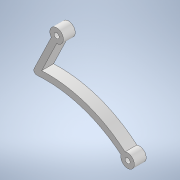
# Autodesk Inventor part: leg_link_3
Saved by Autodesk Inventor 2020 (Build 240168000, 168)
## iProperties
Created: 2020-12-12
Part Number: leg_link_3
Material: Generic
Document SubType Name: Modeling
Designer: Shuang Peng
Density: 1 g/cm^3
Appearance: Default
Author: Shuang Peng
Autodesk Inventor part; units mm, degrees
ref_plane "YZ Plane" through (0, 0, 0) normal (1, 0, 0) x (0, 1, 0)
ref_plane "XZ Plane" through (0, 0, 0) normal (0, 1, 0) x (-1, 0, 0)
ref_plane "XY Plane" through (0, 0, 0) normal (0, 0, 1) x (1, 0, 0)
sketch "Sketch1" plane through (0, 0, 0) normal (0, 0, 1) x (1, 0, 0)
  circle A0 centre (9.3299, 6.9995) radius 4
  line L0 (9.3299, 6.9995) -> (-2.3913, -17.3236)
  circle A1 centre (51.2129, -35.9635) radius 4
  line L1 (9.3299, 6.9995) -> (-2.3913, -17.3236) construction
  line L2 (7.7534, 7.7592) -> (-3.9678, -16.5639)
  line L3 (-0.8148, -18.0833) -> (10.9064, 6.2398)
  arc A2 (10.9064, 6.2398) -> (7.7534, 7.7592) centre (9.3299, 6.9995) ccw
  arc A3 (-3.9678, -16.5639) -> (-0.8148, -18.0833) centre (-2.3913, -17.3236) ccw
  arc A4 (-2.543, -15.5802) -> (-2.2396, -19.067) centre (-2.3913, -17.3236) ccw
  arc A5 (49.9598, -37.1851) -> (52.466, -34.7419) centre (51.2129, -35.9635) ccw
  arc A6 (49.9598, -37.1851) -> (-2.2396, -19.067) centre (2.7702, -88.8875) ccw
  arc A7 (52.466, -34.7419) -> (-2.543, -15.5802) centre (4.0227, -85.2716) ccw
  point P0 (0, 0)
  point P1 (3.4693, -5.1621)
  point P2 (47.3514, -34.9198)
  point P3 (49.7255, -32.2503)
  point P4 (0.4973, -15.3604)
  point P5 (9.3449, 2.9995)
  point P6 (6.1919, 4.5189)
  point P7 (-2.2396, -19.067)
  dimension "d0" = 8
  dimension "d1" = 27
  dimension "d3" = 8
  dimension "d4" = 3.5
  dimension "d6" = 3.5
  dimension "d7" = 70
  dimension "d8" = 70
  constraints: 12 point on circle, 10 end point, 8 centre point, 4 tangent, 2 coincident, 2 equal length, 1 midpoint, 2 other
  measures "d0" diameter of A0
  measures "d1" distance of L0.start L0.end
  measures "d3" diameter of A1
  measures "d4" diameter of A3
  measures "d6" diameter of A5
  measures "d7" radius of A6
  measures "d8" radius of A7
extrude "Extrusion1" add sketch "Sketch1" along normal blind 7
sketch "Sketch2" plane through (0, 0, 7) normal (0, 0, 1) x (1, 0, 0)
  line L0 (0.4973, -15.3604) -> (9.3449, 2.9995) projected
  arc A0 (9.3449, 2.9995) -> (6.1919, 4.5189) centre (9.3299, 6.9995) ccw projected
  line L1 (6.1919, 4.5189) -> (-3.9678, -16.5639) projected
  arc A1 (-3.9678, -16.5639) -> (-2.2396, -19.067) centre (-2.3913, -17.3236) ccw projected
  arc A2 (47.3514, -34.9198) -> (-2.2396, -19.067) centre (2.7702, -88.8875) ccw projected
  arc A3 (47.3514, -34.9198) -> (49.7255, -32.2503) centre (51.2129, -35.9635) ccw projected
  arc A4 (49.7255, -32.2503) -> (0.4973, -15.3604) centre (4.0227, -85.2716) ccw projected
  point P0 (0, 0)
hole "Hole1" at (51.2129, -35.9635, 7) at (9.3299, 6.9995, 7) direction (0, 0, -1) diameter 3 depth 8
sketch "Sketch3" plane through (0, 0, 0) normal (0, 0, -1) x (-1, 0, 0)
  circle A0 centre (-51.2129, -35.9635) radius 1.5 projected
  circle A1 centre (-9.3299, 6.9995) radius 1.5 projected
  line L0 (-0.4973, -15.3604) -> (-9.3449, 2.9995) projected
  arc A2 (-0.4973, -15.3604) -> (-49.7255, -32.2503) centre (-4.0227, -85.2716) ccw projected
  arc A3 (-49.7255, -32.2503) -> (-47.3514, -34.9198) centre (-51.2129, -35.9635) ccw projected
  arc A4 (2.2396, -19.067) -> (-47.3514, -34.9198) centre (-2.7702, -88.8875) ccw projected
  arc A5 (2.2396, -19.067) -> (3.9678, -16.5639) centre (2.3913, -17.3236) ccw projected
  line L1 (-6.1919, 4.5189) -> (3.9678, -16.5639) projected
  arc A6 (-6.1919, 4.5189) -> (-9.3449, 2.9995) centre (-9.3299, 6.9995) ccw projected
  circle A7 centre (-9.3299, 6.9995) radius 4
  circle A8 centre (-51.2129, -35.9635) radius 4
  point P0 (0, 0)
  point P1 (-49.7255, -32.2503)
  dimension "d18" = 8
  dimension "d19" = 8
  constraints: 2 centre point, 2 coincident
  measures "d18" diameter of A7
  measures "d19" diameter of A8
extrude "Extrusion2" cut sketch "Sketch3" against normal blind 2 contours L0 A7 L1 A5 A4 A8 A2
fillet "Fillet1" radius 2 6 edges at (47.3514, -34.9198, 4.5) (48.2239, -33.3053, 2) (49.7255, -32.2503, 4.5) (9.3449, 2.9995, 4.5) (7.5934, 3.3961, 2) (6.1919, 4.5189, 4.5)
body "Solid1"
